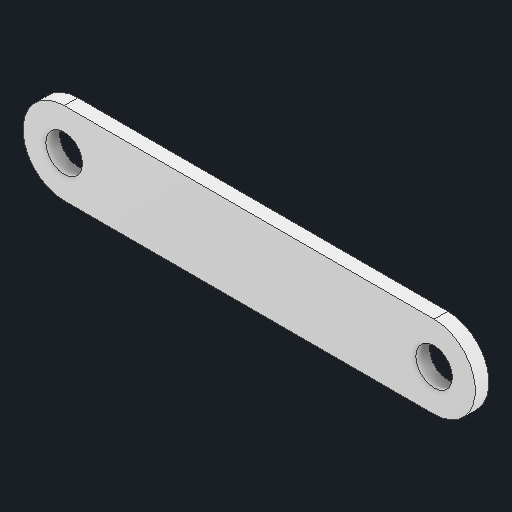
# Autodesk Inventor part: joint_gusset
Saved by Autodesk Inventor 2025 (Build 290162000, 162)
## iProperties
Created: 2024-10-13
Part Number: joint_gusset
Material: Acetal Resin, White
Document SubType Name: Modeling
Designer: Averey Ku
Density: 1.425 g/cm^3
Appearance: Smooth - White
Author: Averey Ku
Autodesk Inventor part; units mm, degrees
ref_plane "YZ Plane" through (0, 0, 0) normal (1, 0, 0) x (0, 1, 0)
ref_plane "XZ Plane" through (0, 0, 0) normal (0, 1, 0) x (-1, 0, 0)
ref_plane "XY Plane" through (0, 0, 0) normal (0, 0, 1) x (1, 0, 0)
sketch "Sketch1" plane through (0, 0, 0) normal (0, 0, 1) x (1, 0, 0)
  circle A0 centre (0, 0) radius 2.1209
  circle A1 centre (42.7862, 0) radius 2.1209
  arc A2 (0, 4.7625) -> (0, -4.7625) centre (0, 0) ccw
  arc A3 (42.7862, -4.7625) -> (42.7862, 4.7625) centre (42.7862, 0) ccw
  line L0 (0, 4.7625) -> (42.7862, 4.7625)
  line L1 (42.7862, -4.7625) -> (0, -4.7625)
  dimension "d0" = 4.2418
  dimension "d1" = 4.2418
  constraints: 4 centre point, 4 end point, 4 point on circle, 3 coincident, 1 horizontal, 1 tangent
  measures "d0" diameter of A0
  measures "d1" diameter of A1
extrude "Extrusion1" add sketch "Sketch1" along normal blind 1.5875
body "Solid1"
